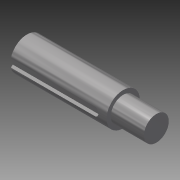
# Autodesk Inventor part: Banebots 0.5x1.5 P60 Shaft
Saved by Autodesk Inventor 2013 (Build 170138000, 138)
## iProperties
Created: 2013-02-18
Part Number: Banebots 0.5x1.5 P60 Shaft
Material: Steel, Carbon
Document SubType Name: Modeling
Designer: Moses
Density: 7.87 g/cm^3
Mass: 41.6527 g
Surface Area: 23.9302 cm^2
Volume: 5.29259 cm^3
Author: Moses
Autodesk Inventor part; units mm, degrees
ref_plane "YZ Plane" through (0, 0, 0) normal (1, 0, 0) x (0, 1, 0)
ref_plane "XZ Plane" through (0, 0, 0) normal (0, 1, 0) x (-1, 0, 0)
ref_plane "XY Plane" through (0, 0, 0) normal (0, 0, 1) x (1, 0, 0)
sketch "Sketch1" plane through (0, 0, 0) normal (1, 0, 0) x (0, 1, 0)
  circle A0 centre (0, 0) radius 6.35
  line L0 (0, 0) -> (0, 6.35) construction
  line L1 (-1.5875, 6.1484) -> (-1.5875, 4.7625)
  line L2 (-1.5875, 4.7625) -> (1.5875, 4.7625)
  line L3 (1.5875, 4.7625) -> (1.5875, 6.1484)
  point P0 (0, 4.7625)
  dimension "d0" = 12.7
  dimension "d2" = 1.5875
  dimension "d3" = 3.175
  constraints: 8 end point, 3 point on circle, 2 parallel, 1 centre point, 1 coincident, 1 midpoint, 1 perpendicular, 1 point on line, 1 vertical
  measures "d0" diameter of A0
  measures "d2" distance from line of L0.end L2
  measures "d3" distance of L1.end L2.end
extrude "Extrusion1" add sketch "Sketch1" along normal blind 38.1
sketch "Sketch2" plane through (38.1, 0, 0) normal (1, 0, 0) x (0, 0, -1)
  circle A0 centre (0, 0) radius 6.35 projected
  circle A1 centre (0, 0) radius 4.7625
  dimension "d6" = 9.525
  constraints: 1 centre point, 1 coincident
  measures "d6" diameter of A1
extrude "Extrusion2" add sketch "Sketch2" along normal blind 12.7 contours A1
extrude "Extrusion3" cut sketch "Sketch1" along normal blind 34.925 contours L3 L2 L1 A0 picked at (0.1781, 5.2842)
fillet "Fillet1" radius 1.5875 2 edges at (34.925, 1.5875, 5.4554) (34.925, -1.5875, 5.4554)
chamfer "Chamfer1" distance 1.27 distance2 2.54 1 edges at (0, 0, -6.35) measured on face at (25.4, -3.3725, 5.3804)
sketch "Sketch3" plane through (0, 0, 0) normal (-1, 0, 0) x (0, 0, 1)
  circle A0 centre (0, 0) radius 3.81 projected
  circle A1 centre (0, 0) radius 2.3495
  dimension "d16" = 4.699
  constraints: 1 centre point, 1 coincident
  measures "d16" diameter of A1
extrude "Extrusion4" cut sketch "Sketch3" against normal blind 12.7 contours A1
thread "Thread1" size "10-32 UNF" class "2B" standard "ANSI Unified Screw Threads" full length
body "Solid1"
